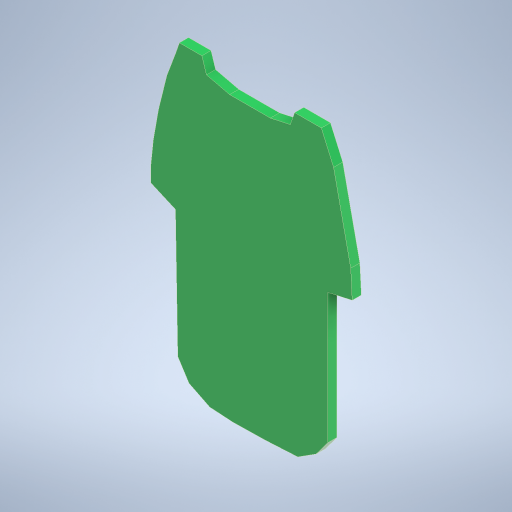
# Autodesk Inventor part: Part2
Saved by Autodesk Inventor 2024 (Build 280153000, 153)
## iProperties
Created: 2024-04-14
Part Number: Part2
Material: Generic
Document SubType Name: Modeling
Designer: Hitesh
Density: 1 g/cm^3
Appearance: Olive Green
Author: Hitesh
Autodesk Inventor part; units mm, degrees
ref_plane "YZ Plane" through (0, 0, 0) normal (1, 0, 0) x (0, 1, 0)
ref_plane "XZ Plane" through (0, 0, 0) normal (0, 1, 0) x (-1, 0, 0)
ref_plane "XY Plane" through (0, 0, 0) normal (0, 0, 1) x (1, 0, 0)
sketch "Sketch1" plane through (0, 0, 0) normal (0, 0, 1) x (1, 0, 0)
  line L0 (26.9534, 140.31) -> (36.8306, 140.31)
  line L1 (36.8306, 140.31) -> (38.8061, 134.065)
  line L2 (38.8061, 134.065) -> (49.002, 131.6435)
  line L3 (49.002, 131.6435) -> (58.0509, 131.6435)
  line L4 (58.0509, 131.6435) -> (66.8448, 131.6435)
  line L5 (66.8448, 131.6435) -> (75.6388, 133.5552)
  line L6 (75.6388, 133.5552) -> (77.526, 139.065)
  line L7 (77.526, 139.065) -> (89.2513, 139.065)
  line L8 (89.2513, 139.065) -> (93.4636, 129.481)
  line L9 (93.4636, 129.481) -> (94.6369, 126.8115)
  line L10 (94.6369, 126.8115) -> (96.9293, 116.2664)
  line L11 (96.9293, 116.2664) -> (99.976, 102.2517)
  line L12 (99.976, 102.2517) -> (102.1542, 92.2318)
  line L13 (102.1542, 92.2318) -> (102.8007, 80.352)
  line L14 (102.8007, 80.352) -> (92.1232, 78.0307)
  line L15 (92.1232, 78.0307) -> (92.1232, 20.902)
  line L16 (92.1232, 20.902) -> (86.9727, 14.0196)
  line L17 (86.9727, 14.0196) -> (78.9304, 8.8886)
  line L18 (78.9304, 8.8886) -> (64.5453, 8.1057)
  line L19 (64.5453, 8.1057) -> (50.4611, 7.8467)
  line L20 (50.4611, 7.8467) -> (40.2944, 8.4971)
  line L21 (40.2944, 8.4971) -> (31.1734, 13.0172)
  line L22 (31.1734, 13.0172) -> (26.2605, 20.7176)
  line L23 (26.2605, 20.7176) -> (25.2413, 76.1313)
  line L24 (25.2413, 76.1313) -> (14.3454, 80.8506)
  line L25 (14.3454, 80.8506) -> (14.3454, 86.7328)
  line L26 (14.3454, 86.7328) -> (15.5218, 97.7359)
  line L27 (15.5218, 97.7359) -> (16.6126, 103.8324)
  line L28 (16.6126, 103.8324) -> (17.7826, 110.3719)
  line L29 (17.7826, 110.3719) -> (21.4653, 125.2093)
  line L30 (21.4653, 125.2093) -> (25.2413, 135.3116)
  line L31 (25.2413, 135.3116) -> (26.9534, 140.31)
  point P0 (0, 0)
  constraints: 64 end point, 6 perpendicular, 5 point on line, 4 parallel, 1 horizontal
extrude "Extrusion1" add sketch "Sketch1" along normal blind 4
body "Solid1"
